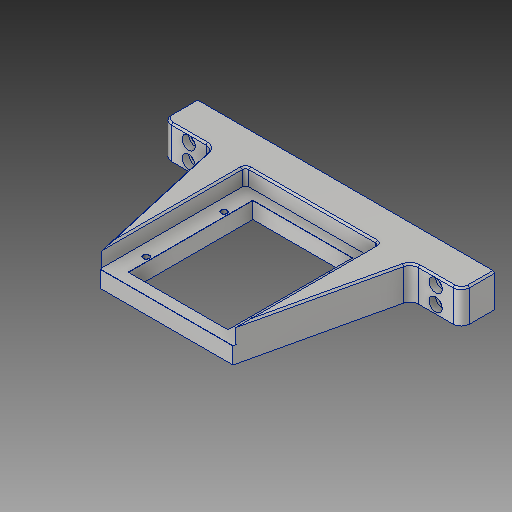
# Autodesk Inventor part: Z-Motorhalter
Saved by Autodesk Inventor 2019 (Build 230136000, 136)
## iProperties
Created: 2021-04-24
Part Number: Z-Motorhalter
Material: Aluminium 6061
Document SubType Name: Modeling
Designer: Michael Sumper
Density: 2.7 g/cm^3
Appearance: Aluminium - flach
Mass: 349.07 g
Surface Area: 320.099 cm^2
Volume: 129.285 cm^3
Author: Michael Sumper
Autodesk Inventor part; units mm, degrees
ref_plane "YZ Plane" through (0, 0, 0) normal (1, 0, 0) x (0, 1, 0)
ref_plane "XZ Plane" through (0, 0, 0) normal (0, 1, 0) x (-1, 0, 0)
ref_plane "XY Plane" through (0, 0, 0) normal (0, 0, 1) x (1, 0, 0)
sketch "Skizze1" plane through (0, 0, 0) normal (0, 1, 0) x (-1, 0, 0)
  line L0 (0, 0) -> (90, 0)
  line L1 (90, 0) -> (90, 20)
  line L2 (90, 20) -> (60, 20)
  line L3 (60, 20) -> (40, 107.7496)
  line L4 (40, 107.7496) -> (-40, 107.7496)
  line L5 (-40, 107.7496) -> (-60, 20)
  line L6 (-60, 20) -> (-90, 20)
  line L7 (-90, 20) -> (-90, 0)
  line L8 (-90, 0) -> (0, 0)
  dimension "d0" = 90
  dimension "d1" = 20
  dimension "d2" = 30
  dimension "d3" = 90
  dimension "d4" = 80
  dimension "d5" = 90
  dimension "d6" = 30
  dimension "d7" = 20
  dimension "d9" = 90
  constraints: 18 end point, 2 parallel, 2 perpendicular, 2 point on line, 1 collinear, 1 horizontal
  measures "d0" distance of L0.start L0.end
  measures "d1" distance of L0.end L1.end
  measures "d2" distance of L1.end L2.end
  measures "d3" distance of L2.end L3.end
  measures "d4" distance of L3.end L4.end
  measures "d5" distance of L4.end L5.end
  measures "d6" distance of L5.end L6.end
  measures "d7" distance of L6.end L7.end
  measures "d9" distance of L0.start L7.end
extrude "Extrusion1" add sketch "Skizze1" along normal blind 20
sketch "Skizze2" plane through (0, 20, 0) normal (0, 1, 0) x (1, 0, 0)
  line L0 (-60, -20) -> (-40, -107.7496) construction
  line L1 (-60, -20) -> (60, -20) construction
  line L2 (40.25, -107.7998) -> (-40.25, -107.7998)
  line L3 (-40.25, -107.7998) -> (-40.25, -19.9498)
  line L4 (-40.25, -19.9498) -> (40.25, -19.9498)
  line L5 (40.25, -19.9498) -> (40.25, -107.7998)
  line L6 (40.25, -107.7998) -> (-40.25, -19.9498) construction
  line L7 (-40.25, -107.7998) -> (40.25, -19.9498) construction
  point P0 (0, 0)
  point P1 (0, -63.8748)
  point P2 (0, -63.8748)
  dimension "d12" = 80.5
  dimension "d13" = 87.85
  constraints: 14 end point, 3 midpoint, 2 horizontal, 2 parallel, 1 perpendicular, 1 other
  measures "d12" distance of L3.end L4.end
  measures "d13" distance of L2.end L3.end
extrude "Extrusion2" cut sketch "Skizze2" against normal blind 10
sketch "Skizze3" plane through (0, 10, 0) normal (0, 1, 0) x (1, 0, 0)
  line L0 (40.25, -106.6528) -> (40, -107.7496) projected
  line L1 (40.25, -19.9498) -> (40.25, -106.6528) projected
  line L2 (-40.25, -19.9498) -> (40.25, -19.9498) projected
  line L3 (-40.25, -106.6528) -> (-40.25, -19.9498) projected
  line L4 (-40, -107.7496) -> (-40.25, -106.6528) projected
  line L5 (40, -107.7496) -> (-40, -107.7496) projected
  line L6 (30, -25.8013) -> (30, -100.8013)
  line L7 (30, -100.8013) -> (-30, -100.8013)
  line L8 (-30, -100.8013) -> (-30, -25.8013)
  line L9 (-30, -25.8013) -> (30, -25.8013)
  line L10 (30, -25.8013) -> (-30, -100.8013) construction
  line L11 (30, -100.8013) -> (-30, -25.8013) construction
  line L12 (-32.75, -100.2496) -> (-32.75, -27.4498) construction
  line L13 (-32.75, -27.4498) -> (32.75, -27.4498) construction
  line L14 (32.75, -27.4498) -> (32.75, -100.2496) construction
  line L15 (32.75, -100.2496) -> (-32.75, -100.2496) construction
  line L16 (-32.75, -63.8497) -> (-32.75, -40.3497) construction
  line L17 (-32.75, -63.8497) -> (-32.75, -87.3497) construction
  line L18 (-32.75, -87.3497) -> (32.75, -87.3497) construction
  line L19 (-32.75, -40.3497) -> (32.75, -40.3497) construction
  circle A0 centre (-32.75, -87.3497) radius 1.75
  circle A1 centre (-32.75, -40.3497) radius 1.75
  circle A2 centre (32.75, -40.3497) radius 1.75
  circle A3 centre (32.75, -87.3497) radius 1.75
  point P0 (0, 0)
  point P1 (0, -63.3013)
  point P2 (0, -63.3013)
  dimension "d16" = 75
  dimension "d17" = 60
  dimension "d18" = 7.5
  dimension "d19" = 23.5
  dimension "d20" = 23.5
  dimension "d21" = 3.5
  dimension "d22" = 3.5
  dimension "d23" = 3.5
  dimension "d24" = 3.5
  constraints: 28 end point, 4 centre point, 4 coincident, 4 midpoint, 4 point on line, 3 perpendicular, 2 parallel, 1 vertical, 4 other
  measures "d16" distance of L6.start L6.end
  measures "d17" distance of L6.end L7.end
  measures "d18" distance between parallel lines of L5 L15
  measures "d19" distance of L16.start L16.end
  measures "d20" distance of L16.start L17.end
  measures "d21" diameter of A0
  measures "d22" diameter of A1
  measures "d23" diameter of A2
  measures "d24" diameter of A3
extrude "Extrusion3" cut sketch "Skizze3" against normal blind 10 contours L6 L7 L8 L9 | A0 | A1 | A2 | A3
fillet "Rundung1" radius 5 4 edges at (-90, 10, 20) (90, 10, 20) (60, 10, 20) (-60, 10, 20)
fillet "Rundung2" radius 2 2 edges at (-40.25, 15, 19.9498) (40.25, 15, 19.9498)
sketch "Skizze4" plane through (-85, 0, 20) normal (0, 0, 1) x (1, 0, 0)
  line L0 (21.0114, 20) -> (21.0114, 0) construction
  line L1 (0, 20) -> (21.0114, 20) construction
  line L2 (0, 0) -> (0, 20) construction
  line L3 (0, 0) -> (21.0114, 0) construction
  line L4 (0, 0) -> (0, 20) construction
  line L5 (148.9886, 0) -> (148.9886, 20) construction
  line L6 (148.9886, 0) -> (170, 0) construction
  line L7 (170, 20) -> (170, 0) construction
  line L8 (148.9886, 20) -> (170, 20) construction
  line L9 (175, 20) -> (-5, 20) construction
  line L10 (159.4943, 20) -> (159.4943, 0) construction
  line L11 (148.9886, 10) -> (170, 10) construction
  line L12 (170, 20) -> (170, 0) construction
  line L13 (148.9886, 10) -> (159.4943, 20) construction
  line L14 (148.9886, 0) -> (148.9886, 20) construction
  line L15 (148.9886, 20) -> (159.4943, 10) construction
  line L16 (154.2415, 15) -> (159.4943, 15) construction
  line L17 (148.9886, 10) -> (159.4943, 0) construction
  line L18 (159.4943, 10) -> (148.9886, 0) construction
  line L19 (154.2415, 5) -> (159.4943, 5) construction
  line L20 (10.5057, 20) -> (10.5057, 0) construction
  line L21 (0, 20) -> (10.5057, 10) construction
  line L22 (10.5057, 20) -> (0, 10) construction
  line L23 (0, 10) -> (10.5057, 0) construction
  line L24 (10.5057, 10) -> (0, 0) construction
  line L25 (5.2528, 5) -> (10.5057, 5) construction
  line L26 (5.2528, 15) -> (10.5057, 15) construction
  point P0 (85, 0)
  constraints: 30 end point, 11 midpoint, 7 point on line, 4 parallel, 4 perpendicular
hole "Bohrung1" at (74.4943, 15, 20) at (74.4943, 5, 20) at (-74.4943, 15, 20) at (-74.4943, 5, 20) direction (0, 0, -1) diameter 4.5 end through all counterbore diameter 8 counterbore depth 4 clearance for "Innensechskantkopfschraube" size "M4" standard "ANSI Metrisches M Profil"
chamfer "Fase1" distance 0.1 angle 45 8 edges at (-30, 10, 63.3013) (0, 10, 25.8013) (0, 10, 100.8013) (30, 10, 63.3013) (31, 10, 40.3497) (31, 10, 87.3497) (-34.5, 10, 40.3497) (-34.5, 10, 87.3497)
chamfer "Fase2" distance 1 angle 45 15 edges at (-40.25, 20, 64.3013) (-39.6642, 20, 20.5356) (0, 20, 19.9498) (39.6642, 20, 20.5356) (40.25, 20, 64.3013) (-49.6818, 20, 65.2708) (-60.8706, 20, 21.0913) (-74.4943, 20, 20) (-88.5355, 20, 18.5355) (-90, 20, 7.5) (49.6818, 20, 65.2708) (60.8706, 20, 21.0913) (74.4943, 20, 20) (88.5355, 20, 18.5355) (90, 20, 7.5)
chamfer "Fase3" distance 0.1 angle 45 1 edges at (0, 10, 107.7496)
thread "Gewinde1" size "M3x0.5" class "6H" standard "ANSI Metric M Profile" full length
thread "Gewinde2" size "M3x0.5" class "6H" standard "ANSI Metric M Profile" full length
thread "Gewinde3" size "M3x0.5" class "6H" standard "ANSI Metric M Profile" full length
thread "Gewinde4" size "M3x0.5" class "6H" standard "ANSI Metric M Profile" full length
